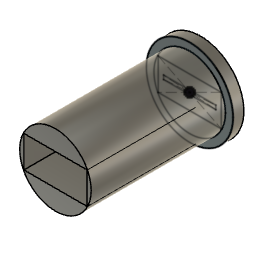
bouchon pilowtech v1 (Autodesk Fusion 360 design; units mm, degrees)
Autodesk Fusion 360 part; units mm, degrees
sketch "Esquisse1" plane through (0, 0, 0) normal (0, 1, 0) x (1, 0, 0)
  circle A0 centre (0, 0) radius 20
  circle A1 centre (0, 0) radius 16.5
  line L0 (12.05, 0.9) -> (-12.05, 0.9)
  line L1 (-12.05, 0.9) -> (-12.05, -0.9)
  line L2 (-12.05, -0.9) -> (12.05, -0.9)
  line L3 (12.05, -0.9) -> (12.05, 0.9)
  line L4 (12.05, 0.9) -> (-12.05, -0.9) construction
  line L5 (-12.05, 0.9) -> (12.05, -0.9) construction
  line L6 (14.55, -7.3) -> (-14.55, -7.3)
  line L7 (-14.55, -7.3) -> (-14.55, 7.3)
  line L8 (-14.55, 7.3) -> (14.55, 7.3)
  line L9 (14.55, 7.3) -> (14.55, -7.3)
  line L10 (14.55, -7.3) -> (-14.55, 7.3) construction
  line L11 (-14.55, -7.3) -> (14.55, 7.3) construction
  dimension "d1" = 40
  dimension "d2" = 33
  dimension "d3" = 24.1
  dimension "d4" = 1.8
  dimension "d6" = 29.1
  dimension "d7" = 14.6
  constraint coincident A0.centre A1.centre
  constraint concentric A0 A1
  constraint horizontal L0
  constraint perpendicular L0 L1
  constraint parallel L0 L2
  constraint parallel L1 L3
  constraint coincident L4 A0.centre
  constraint coincident L5 A0.centre
  constraint horizontal L6
  constraint perpendicular L6 L7
  constraint parallel L6 L8
  constraint parallel L7 L9
  constraint coincident L10 A0.centre
  constraint coincident L11 A0.centre
  measures "d1" diameter of A0
  measures "d2" diameter of A1
  measures "d3" distance of L1.end L2.end
  measures "d4" distance of L0.end L1.end
  measures "d6" distance of L7.end L8.end
  measures "d7" distance of L6.end L7.end
extrude "Extrusion1" add sketch "Esquisse1" along normal blind 5 contours A0 | A1 | L6 L7 L8 L9
extrude "Extrusion2" add sketch "Esquisse1" against normal blind 12 contours A1 | L6 L7 L8 L9
extrude "Extrusion3" add sketch "Esquisse1" against normal blind 62 contours A1
equation "d3 = 23.9 mm + err"
equation "d4 = 1.6 mm + ( err )"
equation "err = 0.2 mm" comment "erreur de l'impression"
equation "d6 = 28.9 mm + err"
equation "d7 = 14.4 mm + err"
equation "d12 = -12 mm - 50 mm"
